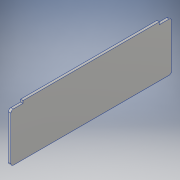
# Autodesk Inventor part: sides
Saved by Autodesk Inventor 2018.1 (Build 221171000, 171)
## iProperties
Created: 2018-11-08
Part Number: sides
Material: Aluminum 6061
Document SubType Name: Sheet Metal
Designer: RCCol
Density: 2.7 g/cm^3
Sheet Metal Rule: .125 thick aluminum
Appearance: Aluminum - Flat
Author: RCCol
Autodesk Inventor part; units mm, degrees
ref_plane "YZ Plane" through (0, 0, 0) normal (1, 0, 0) x (0, 1, 0)
ref_plane "XZ Plane" through (0, 0, 0) normal (0, 1, 0) x (-1, 0, 0)
ref_plane "XY Plane" through (0, 0, 0) normal (0, 0, 1) x (1, 0, 0)
sketch "Sketch1" plane through (0, 0, 0) normal (1, 0, 0) x (0, 1, 0)
  line L0 (63.5, -15.875) -> (63.5, -3.175)
  arc A0 (63.5, -3.175) -> (60.325, 0) centre (60.325, -3.175) ccw
  line L1 (60.325, 0) -> (3.175, 0)
  arc A1 (3.175, 0) -> (0, -3.175) centre (3.175, -3.175) ccw
  line L2 (0, -3.175) -> (0, -206.375)
  arc A2 (0, -206.375) -> (3.175, -209.55) centre (3.175, -206.375) ccw
  line L3 (3.175, -209.55) -> (60.325, -209.55)
  arc A3 (60.325, -209.55) -> (63.5, -206.375) centre (60.325, -206.375) ccw
  line L4 (63.5, -206.375) -> (63.5, -193.675)
  line L5 (63.5, -193.675) -> (66.675, -193.675)
  line L6 (66.675, -193.675) -> (66.675, -15.875)
  line L7 (66.675, -15.875) -> (63.5, -15.875)
  line L8 (63.5, -3.175) -> (63.5, -15.875)
  line L9 (63.5, -193.675) -> (66.675, -193.675)
  line L10 (63.5, -193.675) -> (63.5, -206.375)
  line L11 (60.325, -209.55) -> (3.175, -209.55)
  line L12 (0, -206.375) -> (0, -3.175)
  arc A4 (63.5, -3.175) -> (60.325, 0) centre (60.325, -3.175) ccw
  arc A5 (3.175, 0) -> (0, -3.175) centre (3.175, -3.175) ccw
  point P0 (0, 0)
extrude "Plate1" add sketch "Sketch1" along normal blind 3.175
equation "\"d0\" = Thickness"
equation "\"BendRadius\" = Thickness"
equation "\"BendReliefWidth\" = Thickness"
equation "\"BendReliefDepth\" = 0.5 * Thickness"
equation "\"CornerReliefSize\" = 4 * Thickness"
equation "\"MinimumRemnant\" = 2 * Thickness"
equation "\"TransitionRadius\" = BendRadius"
equation "\"JacobiRadiusSize\" = BendRadius"
equation "\"GapSize\" = Thickness"
equation "\"Thickness\" = 3.175"
body "Solid1"
